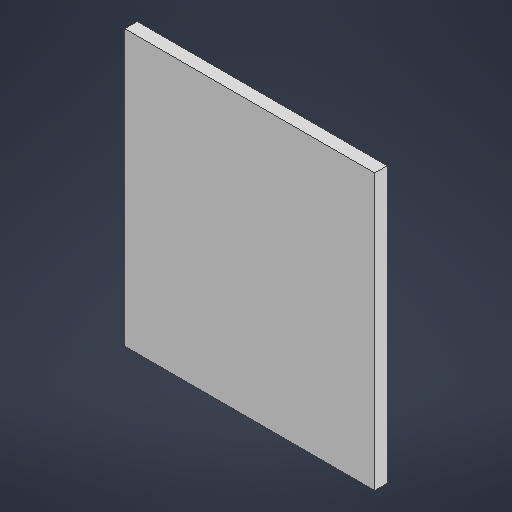
# Autodesk Inventor part: base
Saved by Autodesk Inventor 2026.2 (Build 302298000, 298)
## iProperties
Created: 2026-02-23
Part Number: base
Material: Generic
Document SubType Name: Modeling
Designer: danda
Density: 1 g/cm^3
Appearance: Default
Author: danda
Autodesk Inventor part; units mm, degrees
ref_plane "YZ Plane" through (0, 0, 0) normal (1, 0, 0) x (0, 1, 0)
ref_plane "XZ Plane" through (0, 0, 0) normal (0, 1, 0) x (-1, 0, 0)
ref_plane "XY Plane" through (0, 0, 0) normal (0, 0, 1) x (1, 0, 0)
sketch "Sketch1" plane through (0, 0, 0) normal (0, 0, 1) x (1, 0, 0)
  line L0 (-94.1226, 146.9917) -> (105.8774, 146.9917)
  line L1 (105.8774, 146.9917) -> (105.8774, -73.0083)
  line L2 (105.8774, -73.0083) -> (-94.1226, -73.0083)
  line L3 (-94.1226, -73.0083) -> (-94.1226, 146.9917)
  point P0 (0, 0)
  dimension "d0" = 200
  dimension "d1" = 220
  constraints: 8 end point, 2 parallel, 1 horizontal, 1 perpendicular
  measures "d0" distance of L1.end L2.end
  measures "d1" distance of L0.end L1.end
extrude "Extrusion1" add sketch "Sketch1" along normal blind 10
body "Solid1"
